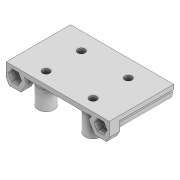
# Autodesk Inventor part: Palm Spacer
Saved by Autodesk Inventor 2021 (Build 250183000, 183)
## iProperties
Created: 2022-09-22
Part Number: Palm Spacer
Material: Generic
Document SubType Name: Modeling
Designer: ereg140
Density: 1 g/cm^3
Appearance: Default
Author: ereg140
Autodesk Inventor part; units mm, degrees
ref_plane "YZ Plane" through (0, 0, 0) normal (1, 0, 0) x (0, 1, 0)
ref_plane "XZ Plane" through (0, 0, 0) normal (0, 1, 0) x (-1, 0, 0)
ref_plane "XY Plane" through (0, 0, 0) normal (0, 0, 1) x (1, 0, 0)
sketch "Sketch1" plane through (0, 0, 0) normal (0, 1, 0) x (-1, 0, 0)
  line L0 (17.5625, -11.9) -> (-17.5625, -11.9)
  line L1 (-17.5625, -11.9) -> (-17.5625, 10)
  line L2 (-17.5625, 10) -> (17.5625, 10)
  line L3 (17.5625, 10) -> (17.5625, -11.9)
  circle A0 centre (8, -6) radius 1.25
  circle A1 centre (-8, -6) radius 1.25
  circle A2 centre (8, 6) radius 1.25
  circle A3 centre (-8, 6) radius 1.25
  point P0 (0, 0)
  point P1 (0, -11.9)
  dimension "d1" = 2.5
  dimension "d2" = 2.5
  dimension "d3" = 2.5
  dimension "d4" = 2.5
  dimension "d5" = 5.9
  dimension "d6" = 16
  dimension "d7" = 12
  dimension "d8" = 8
  dimension "d9" = 6
  dimension "d10" = 4
  dimension "d11" = 35.125
  constraints: 8 end point, 4 centre point, 3 vertical alignment, 2 horizontal alignment, 2 parallel, 1 horizontal, 1 midpoint, 1 perpendicular
  measures "d1" diameter of A0
  measures "d2" diameter of A1
  measures "d3" diameter of A2
  measures "d4" diameter of A3
  measures "d5" distance from line of L0 A0.centre
  measures "d6" distance of A1.centre A0.centre
  measures "d7" distance of A0.centre A2.centre
  measures "d8" horizontal distance of point (0, 0) A0.centre
  measures "d9" vertical distance of point (0, 0) A2.centre
  measures "d10" distance from line of A2.centre L2
  measures "d11" distance between parallel lines of L1 L3
extrude "Extrusion1" add sketch "Sketch1" along normal blind 10
sketch "Sketch2" plane through (17.5625, 0, -11.9) normal (0, 0, -1) x (-1, 0, 0)
  circle A0 centre (3, 7) radius 1
  circle A1 centre (32.125, 7) radius 1
  line L0 (0, 10) -> (35.125, 10) projected
  point P0 (17.5625, 0)
  dimension "d14" = 29.125
  dimension "d15" = 14.5625
  dimension "d16" = 2
  dimension "d17" = 2
  dimension "d18" = 3
  constraints: 2 centre point, 1 horizontal alignment
  measures "d14" distance of A1.centre A0.centre
  measures "d15" horizontal distance of point (17.562, 0) A0.centre
  measures "d16" diameter of A0
  measures "d17" diameter of A1
  measures "d18" distance from line of L0 A0.centre
extrude "Extrusion2" cut sketch "Sketch2" against normal through all
sketch "Sketch5" plane through (-17.5625, 0, 10) normal (0, 0, 1) x (1, 0, 0)
  circle A0 centre (3, 7) radius 1 projected
  circle A1 centre (32.125, 7) radius 1 projected
  line L0 (4.1258, 8.95) -> (5.2517, 7)
  line L1 (5.2517, 7) -> (4.1258, 5.05)
  line L2 (4.1258, 5.05) -> (1.8742, 5.05)
  line L3 (1.8742, 5.05) -> (0.7483, 7)
  line L4 (0.7483, 7) -> (1.8742, 8.95)
  line L5 (1.8742, 8.95) -> (4.1258, 8.95)
  line L6 (30.9992, 8.95) -> (33.2508, 8.95)
  line L7 (33.2508, 8.95) -> (34.3767, 7)
  line L8 (34.3767, 7) -> (33.2508, 5.05)
  line L9 (33.2508, 5.05) -> (30.9992, 5.05)
  line L10 (30.9992, 5.05) -> (29.8733, 7)
  line L11 (29.8733, 7) -> (30.9992, 8.95)
  point P0 (17.5625, 0)
  dimension "d25" = 3.9
  dimension "d26" = 3.9
  constraints: 24 end point, 2 coincident, 1 horizontal, 1 point on line, 26 other
  measures "d25" distance between parallel lines of L2 L5
  measures "d26" distance between parallel lines of L6 L9
extrude "Extrusion3" cut sketch "Sketch5" against normal blind 2 contours A0 | A1 | L0 L1 L2 L3 L4 L5 | L6 L7 L8 L9 L10 L11
shell "Shell1" thickness 1.5 removed faces 5 at (-14.7439, 0, -2.4397) at (-17.5625, 3.3333, -4.6) at (-4.6047, 2.1123, -11.9) at (17.5625, 3.3333, 2.7) at (4.4789, 1.6833, 10)
fillet "Fillet1" radius 2 6 edges at (-5.25, 8.5, -6) (-5.5228, 8.5, 7.1942) (-10.4772, 8.5, 4.8058) (9.1942, 8.5, 8.4772) (6.8058, 8.5, 3.5228) (10.75, 8.5, -6)
fillet "Fillet2" [suppressed]
fillet "Fillet3" radius 1 2 edges at (-16.5625, 8.5, -2.7) (16.5625, 8.5, -2.7)
equation "\"d4\" = d2"
equation "\"d8\" = 0.5 * d6"
equation "\"d9\" = 0.5 * d7"
equation "\"d15\" = 0.5 * d14"
body "Solid1"
